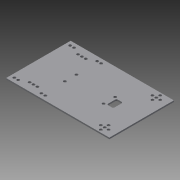
# Autodesk Inventor part: Body
Saved by Autodesk Inventor 2014 SP1 (Build 180222100, 222)
## iProperties
Created: 2014-04-23
Part Number: Body
Material: Generic
Document SubType Name: Modeling
Designer: david
Density: 1 g/cm^3
Appearance: Default
Author: david
Autodesk Inventor part; units mm, degrees
ref_plane "YZ Plane" through (0, 0, 0) normal (1, 0, 0) x (0, 1, 0)
ref_plane "XZ Plane" through (0, 0, 0) normal (0, 1, 0) x (-1, 0, 0)
ref_plane "XY Plane" through (0, 0, 0) normal (0, 0, 1) x (1, 0, 0)
sketch "Sketch1" plane through (0, 0, 0) normal (0, 1, 0) x (-1, 0, 0)
  line L0 (80, -50) -> (-80, -50)
  line L1 (-80, -50) -> (-80, 50)
  line L2 (-80, 50) -> (80, 50)
  line L3 (80, 50) -> (80, -50)
  line L4 (0, 0) -> (0, -16.1308) construction
  line L5 (0, 0) -> (18.4922, 0) construction
  dimension "d1" = 100
  dimension "d2" = 160
  constraints: 12 end point, 3 parallel, 2 perpendicular, 1 horizontal, 2 other
  measures "d1" distance between parallel lines of L0 L2
  measures "d2" distance between parallel lines of L3 L1
extrude "Extrusion1" add sketch "Sketch1" along normal blind 2.2
sketch "Sketch2" plane through (0, 2.2, 0) normal (0, 1, 0) x (1, 0, 0)
  line L0 (-80, -50) -> (80, -50) projected
  line L1 (80, -50) -> (80, 50) projected
  line L2 (80, -50) -> (80, -30)
  line L3 (80, -30) -> (45.6, -30)
  line L4 (45.6, -30) -> (45.6, -50)
  line L5 (45.6, -50) -> (80, -50)
  line L6 (80, -40) -> (45.6, -40) construction
  circle A0 centre (68.8, -40) radius 2.15
  circle A1 centre (62.8, -40) radius 2.15
  circle A2 centre (56.8, -40) radius 2.15
  line L7 (62.8, -40) -> (62.8, -30) construction
  circle A3 centre (62.8, -34) radius 2.15
  circle A4 centre (62.8, -46) radius 2.15
  circle A5 centre (62.8, -40) radius 2.15
  line L8 (0, 0) -> (96.2626, 0) construction
  line L9 (80, 50) -> (80, 30)
  line L10 (80, 30) -> (45.6, 30)
  line L11 (45.6, 30) -> (45.6, 50)
  line L12 (45.6, 50) -> (80, 50)
  line L13 (80, 40) -> (45.6, 40) construction
  circle A6 centre (68.8, 40) radius 2.15
  circle A7 centre (62.8, 40) radius 2.15
  circle A8 centre (56.8, 40) radius 2.15
  line L14 (62.8, 40) -> (62.8, 30) construction
  circle A9 centre (62.8, 34) radius 2.15
  circle A10 centre (62.8, 46) radius 2.15
  circle A11 centre (62.8, 40) radius 2.15
  line L15 (80, 50) -> (-80, 50) projected
  line L16 (-80, 50) -> (-80, -50) projected
  line L17 (-38, 40) -> (-62, 40)
  line L18 (-62, 40) -> (-62, 50)
  line L19 (-62, 50) -> (-38, 50)
  line L20 (-38, 50) -> (-38, 40)
  line L21 (-74.3246, 46.5) -> (-4.1674, 46.5) construction
  line L22 (-50, 53.3324) -> (-50, 32.9187) construction
  circle A12 centre (-50, 37.5) radius 2.15
  line L23 (-68.3246, 46.5) -> (1.8326, 46.5) construction
  circle A13 centre (-44, 37.5) radius 2.15
  circle A14 centre (-56, 37.5) radius 2.15
  line L24 (-8.0003, 43.25) -> (-83.9137, 43.25) construction
  circle A15 centre (-68, 43.25) radius 2.15
  circle A16 centre (-74, 43.25) radius 2.15
  circle A17 centre (-32, 43.25) radius 2.15
  circle A18 centre (-26, 43.25) radius 2.15
  line L25 (-38, -40) -> (-62, -40)
  line L26 (-62, -40) -> (-62, -50)
  line L27 (-62, -50) -> (-38, -50)
  line L28 (-38, -50) -> (-38, -40)
  line L29 (-74.3246, -46.5) -> (-4.1674, -46.5) construction
  line L30 (-50, -53.3324) -> (-50, -32.9187) construction
  circle A19 centre (-50, -37.5) radius 2.15
  circle A20 centre (-44, -37.5) radius 2.15
  circle A21 centre (-56, -37.5) radius 2.15
  line L31 (-8.0003, -43.25) -> (-83.9137, -43.25) construction
  circle A22 centre (-68, -43.25) radius 2.15
  circle A23 centre (-74, -43.25) radius 2.15
  circle A24 centre (-26, -43.25) radius 2.15
  circle A25 centre (-32, -43.25) radius 2.15
  circle A26 centre (-50, 37.5) radius 2.5 construction
  point P0 (80, 50)
  dimension "d13" = 20
  dimension "d14" = 34.4
  dimension "d15" = 4.3
  dimension "d16" = 6
  dimension "d17" = 6
  dimension "d18" = 6
  dimension "d27" = 24
  dimension "d28" = 10
  dimension "d29" = 18
  dimension "d31" = 4.3
  dimension "d34" = 6
  dimension "d41" = 6
  dimension "d46" = 6.5
  dimension "d48" = 4.3
  dimension "d49" = 6
  dimension "d52" = 6
  dimension "d60" = 5
  constraints: 56 end point, 35 symmetric about line, 27 centre point, 10 point on line, 7 parallel, 5 horizontal, 4 midpoint, 4 perpendicular, 3 collinear, 2 vertical, 1 concentric, 1 tangent, 36 other
  measures "d13" distance of L2.start L2.end
  measures "d14" distance of L4.end L2.start
  measures "d15" diameter of A0
  measures "d16" distance of A0.centre L7.start
  measures "d17" distance of L7.start A3.centre
  measures "d18" distance of L7.start A4.centre
  measures "d27" distance between parallel lines of L20 L18
  measures "d28" distance between parallel lines of L15 L17
  measures "d29" distance between parallel lines of L16 L18
  measures "d31" diameter of A12
  measures "d34" distance of A12.centre A13.centre
  measures "d41" distance of A12.centre A14.centre
  measures "d46" distance between parallel lines of L17 L21
  measures "d48" diameter of A15
  measures "d49" distance from line of L18 A15.centre
  measures "d52" distance of A15.centre A16.centre
  measures "d60" diameter of A26
extrude "Holes" cut sketch "Sketch2" against normal through all contours A0 | A1 | A2 | A3 | A4 | A6 | A7 | A8 | A9 | A10 | A12 | A13 | A14 | A15 | A16 | A17 | A18 | A19 | A20 | A21 | A22 | A23 | A24 | A25
sketch "Sketch3" plane through (0, 2.2, 0) normal (0, 1, 0) x (1, 0, 0)
  line L0 (33.5, 13.5) -> (-33.5, 13.5) construction
  line L1 (-33.5, 13.5) -> (-33.5, -13.5) construction
  line L2 (-33.5, -13.5) -> (33.5, -13.5) construction
  line L3 (33.5, -13.5) -> (33.5, 13.5) construction
  line L4 (0, 0) -> (39.98, 0) construction
  line L5 (0, 0) -> (0, 21.0122) construction
  circle A0 centre (30, 9) radius 2.15
  circle A1 centre (30, -9) radius 2.15
  circle A2 centre (-30, 9) radius 2.15
  circle A3 centre (-30, -9) radius 2.15
  line L6 (33.5, 7.5) -> (43.5, 7.5)
  line L7 (43.5, 7.5) -> (43.5, -7.5)
  line L8 (43.5, -7.5) -> (33.5, -7.5)
  line L9 (33.5, -7.5) -> (33.5, 7.5)
  dimension "d61" = 67
  dimension "d62" = 27
  dimension "d63" = 4.3
  dimension "d64" = 3.5
  dimension "d65" = 4.5
  dimension "d68" = 10
  dimension "d69" = 15
  constraints: 20 end point, 4 centre point, 4 parallel, 4 perpendicular, 3 symmetric about line, 2 horizontal, 1 point on line, 6 other
  measures "d61" distance between parallel lines of L3 L1
  measures "d62" distance between parallel lines of L2 L0
  measures "d63" diameter of A0
  measures "d64" distance from line of L3 A0.centre
  measures "d65" distance from line of A0.centre L0
  measures "d68" distance of L6.start L6.end
  measures "d69" distance between parallel lines of L8 L6
extrude "Extrusion4" cut sketch "Sketch3" against normal through all
fillet "Fillet1" radius 2 4 edges at (33.5, 1.1, -7.5) (43.5, 1.1, -7.5) (43.5, 1.1, 7.5) (33.5, 1.1, 7.5)
equation "\"d1\" = BodyWidth"
equation "\"d2\" = BodyLength"
equation "\"d3\" = Depth"
equation "\"d15\" = Holes"
equation "\"d27\" = MotorWidth"
equation "\"d31\" = Holes"
equation "\"d57\" = Depth"
equation "\"BodyWidth\" = 100"
equation "\"BodyLength\" = 160"
equation "\"Holes\" = 4.3"
equation "\"Depth\" = 2.2"
equation "\"d20\" = 4.3"
equation "\"MotorWidth\" = 24"
body "Solid1"
